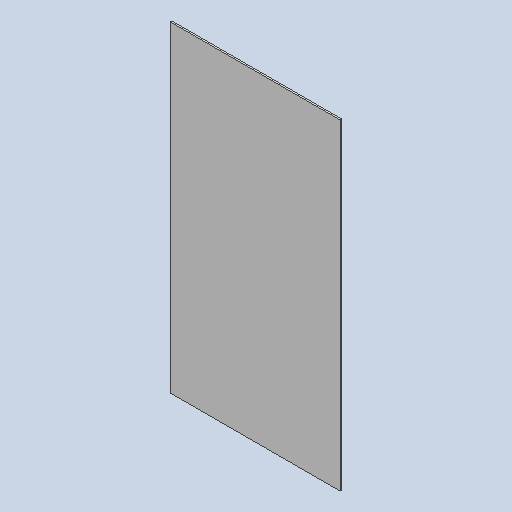
# Autodesk Inventor part: pokrywka
Saved by Autodesk Inventor 2023 (Build 270158000, 158)
## iProperties
Created: 2023-04-06
Part Number: pokrywka
Material: Ogólny
Document SubType Name: Modeling
Designer: Kamil
Density: 1 g/cm^3
Appearance: Domyślna
Author: Kamil
Autodesk Inventor part; units mm, degrees
ref_plane "YZ Plane" through (0, 0, 0) normal (1, 0, 0) x (0, 1, 0)
ref_plane "XZ Plane" through (0, 0, 0) normal (0, 1, 0) x (-1, 0, 0)
ref_plane "XY Plane" through (0, 0, 0) normal (0, 0, 1) x (1, 0, 0)
sketch "Szkic1" plane through (0, 0, 0) normal (0, 0, 1) x (1, 0, 0)
  line L0 (51.6088, -2) -> (51.6088, 5) projected
  line L1 (-0.1391, 5) -> (51.6088, 5) projected
  line L2 (-0.1391, 5) -> (-0.1391, -2) projected
  line L3 (51.6088, -2) -> (-0.1391, -2) projected
  line L4 (51.6088, -86) -> (51.6088, -93) projected
  line L5 (51.6088, -86) -> (-0.1391, -86) projected
  line L6 (-0.1391, -93) -> (-0.1391, -86) projected
  line L7 (-0.1391, -93) -> (51.6088, -93) projected
  line L8 (51.6088, -93) -> (-0.1391, -93)
  line L9 (-0.1391, -93) -> (-0.1391, 5)
  line L10 (-0.1391, 5) -> (51.6088, 5)
  line L11 (51.6088, 5) -> (51.6088, -93)
  circle A0 centre (25.7348, -89.5) radius 1.5 projected
  point P0 (0, 0)
  constraints: 8 end point, 2 parallel, 1 horizontal, 1 perpendicular
extrude "Wyciągnięcie proste1" add sketch "Szkic1" along normal blind 0.5 contours L3 L2 L1 L0 | L11 L5 L9 L3 | L4 L7 L6 L5 | A0
